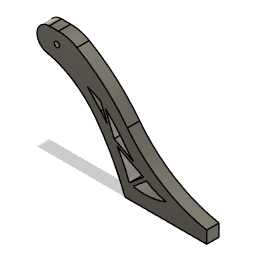
Hinge arm v8 (Autodesk Fusion 360 design; units mm, degrees)
Autodesk Fusion 360 part; units mm, degrees
note: some values were not read from the file. Set by a fixed rule: which sketch regions a step uses.
sketch "Sketch1" plane through (0, 0, 0) normal (0, 0, 1) x (1, 0, 0)
  line L0 (0, 0) -> (50, 0)
  line L1 (50, 0) -> (50, 7.5)
  line L2 (50, 7.5) -> (27.9792, 7.5)
  line L3 (-46.3191, 63.75) -> (-46.3191, 56.25)
  circle A0 centre (-41.6596, 60) radius 1.6
  line L4 (50, 7.5) -> (17.5, 7.5)
  line L5 (-46.3191, 60) -> (-46.3191, 67.5)
  line L6 (-46.3191, 60) -> (-46.3191, 52.5)
  line L7 (-46.3191, 67.5) -> (-35, 67.5)
  line L8 (-46.3191, 52.5) -> (-35.3669, 52.5)
  arc A1 (17.5, 7.5) -> (-35, 67.5) centre (-82.3864, -26.9318) ccw
  arc A2 (0, 0) -> (-35.3669, 52.5) centre (-129.8244, -49.2943) ccw
  dimension "d1" = 50
  dimension "d29" = 3.2
  dimension "d42" = 22.0208
  dimension "d43" = 32.5
  dimension "d50" = 7.5
  dimension "d51" = 7.5
  constraint horizontal L0
  constraint vertical L1
  constraint coincident L0.start A2.start
  constraint vertical L3
  constraint perpendicular L1 L4
  constraint midpoint L3 L5.start
  constraint parallel L3 L5
  constraint parallel L3 L6
  constraint perpendicular L5 L7
  constraint perpendicular L6 L8
  measures "d1" distance of L0.start L0.end
  measures "d29" diameter of A0
  measures "d42" distance of L1.end L2.end
  measures "d43" distance of L1.end L4.end
  measures "d50" distance of L5.start L5.end
  measures "d51" distance of L5.start L6.end
extrude "Extrude1" add sketch "Sketch1" along normal blind 7.5
sketch "Sketch3" plane through (0, 0, 0) normal (0, -1, 0) x (1, 0, 0)
  line L0 (0, 0) -> (50, 0)
  line L1 (50, 0) -> (50, 7.5)
  line L2 (50, 7.5) -> (0, 7.5)
  circle A0 centre (10, 3.75) radius 2.45
  circle A1 centre (25, 3.75) radius 2.45
  circle A2 centre (40, 3.75) radius 2.45
  line L3 (0, 7.5) -> (0, 0)
  dimension "d21" = 4.9
  dimension "d23" = 4.9
  dimension "d24" = 15
  dimension "d25" = 4.9
  dimension "d26" = 15
  measures "d21" diameter of A0
  measures "d23" diameter of A1
  measures "d24" distance of A0.centre A1.centre
  measures "d25" diameter of A2
  measures "d26" distance of A1.centre A2.centre
fillet "Fillet11" radius 79.5 1 edges at (17.5, 7.5, 3.75)
fillet "Fillet12" radius 22.5 1 edges at (-35, 67.5, 3.75)
fillet "Fillet13" radius 52.5 1 edges at (-35.3669, 52.5, 3.75)
extrude "Extrude3" cut sketch "Sketch3" against normal blind 5 contours A0 | A1 | A2
sketch "Sketch5" plane through (0, 0, 7.5) normal (0, 0, 1) x (1, 0, 0)
  line L0 (-46.3191, 67.5) -> (-46.3191, 52.5)
  line L1 (0, 0) -> (50, 0)
  line L2 (50, 0) -> (50, 7.5)
  circle A0 centre (-41.6596, 60) radius 1.6
  arc A1 (1.4949, 37.3081) -> (-29.3793, 64.4634) centre (-82.3864, -26.9318) ccw
  line L3 (-40.6676, 67.5) -> (-46.3191, 67.5)
  arc A2 (0, 0) -> (-17.9609, 32.991) centre (-129.8244, -49.2943) ccw
  arc A3 (-29.3793, 64.4634) -> (-40.6676, 67.5) centre (-40.6676, 45) ccw
  arc A4 (-17.9609, 32.991) -> (-46.3191, 52.5) centre (-60.2517, 1.8825) ccw
  arc A5 (1.4949, 37.3081) -> (50, 7.5) centre (64.6117, 85.6457) ccw
  arc A6 (1.0424, 26.2196) -> (-11.9, 40.7459) centre (-79.3108, -32.3435) ccw
  arc A7 (5.0466, 8.1893) -> (25, 10) centre (12.1035, 41.2705) ccw
  arc A8 (-14.8041, 38.1437) -> (-23, 47) centre (-327.3726, -242.8958) ccw
  arc A9 (-14.8041, 43.3212) -> (-23, 47) centre (-36.6681, 5.5799) ccw
  line L4 (-14.8041, 43.3212) -> (-10.8744, 33.4524)
  line L5 (-11.9, 40.7459) -> (-6.6314, 27.5143)
  arc A10 (2.6113, 8.8042) -> (-4.75, 24.5019) centre (-79.732, -20.2349) ccw
  arc A11 (-10.8744, 33.4524) -> (-14.8041, 38.1437) centre (-79.732, -20.2349) ccw
  line L6 (-6.6314, 27.5143) -> (5.0466, 21.4896)
  line L7 (-4.75, 24.5019) -> (11.3229, 16.2098)
  line L8 (2.6113, 8.8042) -> (11.3229, 16.2098)
  line L9 (5.0466, 8.1893) -> (13.1098, 15.0439)
  arc A12 (1.0424, 26.2196) -> (5.0466, 21.4896) centre (35.5271, 51.3528) ccw
  arc A13 (13.1098, 15.0439) -> (25, 10) centre (35.5271, 51.3528) ccw
  constraint tangent A1 A6
  constraint tangent A6 A12
  constraint tangent A6 A10
  constraint tangent A8 A10
  constraint coincident L4.end A10
  constraint parallel L4 L5
  constraint concentric A10 A11
  constraint coincident L7.end A12
  constraint parallel L6 L7
  constraint coincident L9.end A12
  constraint parallel L8 L9
  constraint concentric A12 A13
extrude "Extrude4" cut sketch "Sketch5" against normal blind 23 contours A6 L5 L6 A12 | A7 L9 A13 | A8 A9 L4 A11 | A10 L7 L8
sketch "Sketch6" plane through (0, 0, 7.5) normal (0, 0, 1) x (1, 0, 0)
  line L0 (11.3229, 16.2098) -> (2.6113, 8.8042)
  arc A0 (2.6113, 8.8042) -> (-4.75, 24.5019) centre (-79.732, -20.2349) ccw
  line L1 (-4.75, 24.5019) -> (11.3229, 16.2098)
  line L2 (5.0466, 21.4896) -> (-6.6314, 27.5143)
  line L3 (-6.6314, 27.5143) -> (-11.9, 40.7459)
  arc A1 (1.0424, 26.2196) -> (-11.9, 40.7459) centre (-79.3108, -32.3435) ccw
  arc A2 (1.0424, 26.2196) -> (5.0466, 21.4896) centre (35.5271, 51.3528) ccw
  arc A3 (13.1098, 15.0439) -> (25, 10) centre (35.5271, 51.3528) ccw
  arc A4 (5.0466, 8.1893) -> (25, 10) centre (12.1035, 41.2705) ccw
  line L4 (5.0466, 8.1893) -> (13.1098, 15.0439)
  arc A5 (-14.8041, 38.1437) -> (-23, 47) centre (-327.3726, -242.8958) ccw
  arc A6 (-14.8041, 43.3212) -> (-23, 47) centre (-36.6681, 5.5799) ccw
  line L5 (-14.8041, 43.3212) -> (-10.8744, 33.4524)
  arc A7 (-10.8744, 33.4524) -> (-14.8041, 38.1437) centre (-79.732, -20.2349) ccw
  arc A8 (-29.3793, 64.4634) -> (-40.6676, 67.5) centre (-40.6676, 45) ccw
  line L6 (-40.6676, 67.5) -> (-46.3191, 67.5)
  line L7 (-46.3191, 67.5) -> (-46.3191, 52.5)
  arc A9 (-17.9609, 32.991) -> (-46.3191, 52.5) centre (-60.2517, 1.8825) ccw
  arc A10 (0, 0) -> (-17.9609, 32.991) centre (-129.8244, -49.2943) ccw
  line L8 (0, 0) -> (50, 0)
  line L9 (50, 0) -> (50, 7.5)
  arc A11 (1.4949, 37.3081) -> (50, 7.5) centre (64.6117, 85.6457) ccw
  arc A12 (1.4949, 37.3081) -> (-29.3793, 64.4634) centre (-82.3864, -26.9318) ccw
  circle A13 centre (-41.6596, 60) radius 1.6
  arc A14 (-46.3191, 67.5) -> (-46.3191, 52.5) centre (-46.3191, 60) ccw
  constraint midpoint L7 A14.centre
extrude "Extrude5" add sketch "Sketch6" against normal blind 7.5 contours L7 A14
fillet "Fillet14" radius 36.5 1 edges at (-46.3191, 52.5, 3.75)
